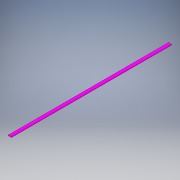
# Autodesk Inventor part: isolation
Saved by Autodesk Inventor 2016 SP1 (Build 200210100, 210)
## iProperties
Created: 2017-07-05
Part Number: isolation
Material: Типовые
Document SubType Name: Modeling
Designer: user
Density: 1 g/cm^3
Appearance: По умолчанию
Author: user
Autodesk Inventor part; units mm, degrees
ref_plane "YZ Plane" through (0, 0, 0) normal (1, 0, 0) x (0, 1, 0)
ref_plane "XZ Plane" through (0, 0, 0) normal (0, 1, 0) x (-1, 0, 0)
ref_plane "XY Plane" through (0, 0, 0) normal (0, 0, 1) x (1, 0, 0)
sketch "Эскиз1" plane through (0, 0, 0) normal (0, 1, 0) x (-1, 0, 0)
  line L0 (18.7, 4.8) -> (-18.7, 4.8)
  line L1 (-23.5, 0) -> (-23.5, 0)
  line L2 (-18.7, -4.8) -> (18.7, -4.8)
  line L3 (23.5, 0) -> (23.5, 0)
  arc A0 (23.5, 0) -> (18.7, 4.8) centre (18.7, 0) ccw
  arc A1 (18.7, -4.8) -> (23.5, 0) centre (18.7, 0) ccw
  arc A2 (-18.7, 4.8) -> (-23.5, 0) centre (-18.7, 0) ccw
  arc A3 (-23.5, 0) -> (-18.7, -4.8) centre (-18.7, 0) ccw
  line L4 (18.7, 4.4) -> (-18.7, 4.4)
  line L5 (-23.1, 0) -> (-23.1, 0)
  line L6 (-18.7, -4.4) -> (18.7, -4.4)
  line L7 (23.1, 0) -> (23.1, 0)
  arc A4 (23.1, 0) -> (18.7, 4.4) centre (18.7, 0) ccw
  arc A5 (18.7, -4.4) -> (23.1, 0) centre (18.7, 0) ccw
  arc A6 (-23.1, 0) -> (-18.7, -4.4) centre (-18.7, 0) ccw
  arc A7 (-18.7, 4.4) -> (-23.1, 0) centre (-18.7, 0) ccw
  point P0 (0, 0)
  dimension "d0" = 4.8
  dimension "d1" = 4.8
  dimension "d2" = 47
  dimension "d3" = 23.5
  dimension "d4" = 4.8
  dimension "d5" = 4.4
  dimension "d6" = 4.4
  dimension "d7" = 23.1
  dimension "d8" = 23.1
  dimension "d9" = 4.4
  constraints: 16 end point, 16 point on circle, 16 tangent, 8 centre point, 6 equal radius, 4 parallel, 2 horizontal, 2 perpendicular
  measures "d0" distance from line of point (0, 0) L0
  measures "d1" distance from line of L2 point (0, 0)
  measures "d2" distance between parallel lines of L1 L3
  measures "d3" distance from line of point (0, 0) L3
  measures "d4" radius of A0
  measures "d5" distance from line of point (0, 0) L4
  measures "d6" distance from line of point (0, 0) L6
  measures "d7" distance from line of L5 point (0, 0)
  measures "d8" distance from line of point (0, 0) L7
  measures "d9" radius of A4
extrude "Выдавливание1" add sketch "Эскиз1" along normal blind 2000
